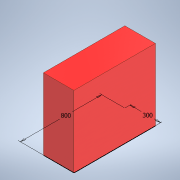
# Autodesk Inventor part: 桌1
Saved by Autodesk Inventor 2022 (Build 260153000, 153)
## iProperties
Created: 2023-03-07
Part Number: 桌1
Material: 一般
Document SubType Name: Modeling
Designer: robot
Density: 1 g/cm^3
Appearance: 銅 - 緞
Mass: 168000 g
Surface Area: 20200 cm^2
Volume: 168000 cm^3
Author: robot
Autodesk Inventor part; units mm, degrees
ref_plane "YZ Plane" through (0, 0, 0) normal (1, 0, 0) x (0, 1, 0)
ref_plane "XZ Plane" through (0, 0, 0) normal (0, 1, 0) x (-1, 0, 0)
ref_plane "XY Plane" through (0, 0, 0) normal (0, 0, 1) x (1, 0, 0)
sketch "草圖1" plane through (0, 0, 0) normal (0, 1, 0) x (-1, 0, 0)
  line L0 (0, 0) -> (300, 0)
  line L1 (300, -800) -> (0, -800)
  line L2 (300, -800) -> (300, 0)
  line L3 (0, -800) -> (0, 0)
  line L4 (300, 0) -> (0, 0)
  dimension "d7" = 300
  dimension "d8" = 800
  constraints: 10 end point, 1 collinear, 1 horizontal, 1 perpendicular, 1 vertical
  measures "d7" distance of L1.start L1.end
  measures "d8" distance of L1.start L0.end
extrude "擠出1" add sketch "草圖1" along normal blind 700
